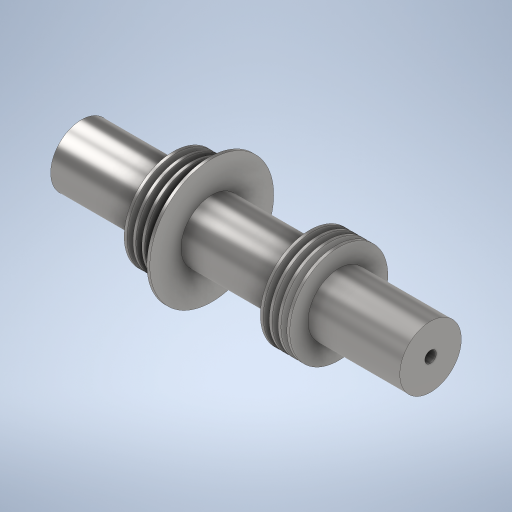
# Autodesk Inventor part: Полный ротор
Saved by Autodesk Inventor 2023 (Build 270158000, 158)
## iProperties
Created: 2023-05-19
Part Number: Полный ротор
Material: Сталь нержавеющая, 440C
Document SubType Name: Modeling
Designer: Roma
Density: 7.75 g/cm^3
Appearance: С умеренной полировкой
Mass: 5.75155e+06 g
Surface Area: 129986 cm^2
Volume: 742136 cm^3
Author: Roma
Autodesk Inventor part; units mm, degrees
ref_plane "YZ Plane" through (0, 0, 0) normal (1, 0, 0) x (0, 1, 0)
ref_plane "XZ Plane" through (0, 0, 0) normal (0, 1, 0) x (-1, 0, 0)
ref_plane "XY Plane" through (0, 0, 0) normal (0, 0, 1) x (1, 0, 0)
derived "Rotor.ipt"
sketch "Эскиз1" plane through (0, 0, 0) normal (0, 0, 1) x (1, 0, 0)
  line L0 (0, 0) -> (3099.5877, 0)
  line L1 (0, 268) -> (800, 268)
  line L2 (800, 268) -> (800, 427.5)
  line L3 (800, 427.5) -> (825.2848, 427.5)
  line L4 (825.2848, 427.5) -> (825.2848, 268)
  line L5 (825.2848, 268) -> (876.9914, 268)
  line L6 (876.9914, 268) -> (876.9914, 427.5)
  line L7 (876.9914, 427.5) -> (902.2762, 427.5)
  line L8 (902.2762, 427.5) -> (902.2762, 268)
  line L9 (902.2762, 268) -> (953.9828, 268)
  line L10 (953.9828, 268) -> (953.9828, 427.5)
  line L11 (953.9828, 427.5) -> (979.2676, 427.5)
  line L12 (979.2676, 427.5) -> (979.2676, 268)
  line L13 (979.2676, 268) -> (1030.9742, 268)
  line L14 (1030.9742, 268) -> (1110.9742, 268)
  line L15 (1110.9742, 268) -> (1110.9742, 540)
  line L16 (1110.9742, 540) -> (1136.259, 540)
  line L17 (1136.259, 540) -> (1136.259, 268)
  line L18 (1136.259, 268) -> (1936.259, 268)
  line L19 (1936.259, 268) -> (1987.9655, 268)
  line L20 (1987.9655, 268) -> (1987.9655, 427.5)
  line L21 (1987.9655, 427.5) -> (2013.2504, 427.5)
  line L22 (2013.2504, 427.5) -> (2013.2504, 268)
  line L23 (2013.2504, 268) -> (2064.9569, 268)
  line L24 (2064.9569, 268) -> (2064.9569, 427.5)
  line L25 (2064.9569, 427.5) -> (2090.2418, 427.5)
  line L26 (2090.2418, 427.5) -> (2090.2418, 268)
  line L27 (2090.2418, 268) -> (2141.9483, 268)
  line L28 (2141.9483, 268) -> (2141.9483, 427.5)
  line L29 (2141.9483, 427.5) -> (2167.2331, 427.5)
  line L30 (2167.2331, 427.5) -> (2167.2331, 268)
  line L31 (2167.2331, 268) -> (2218.9397, 268)
  line L32 (2218.9397, 268) -> (2218.9397, 427.5)
  line L33 (2218.9397, 427.5) -> (2244.2245, 427.5)
  line L34 (2244.2245, 427.5) -> (2244.2245, 268)
  line L35 (2244.2245, 268) -> (3044.2245, 268)
  line L36 (0, 50) -> (3044.2245, 50)
  line L37 (3044.2245, 50) -> (3044.2245, 268)
  line L38 (0, 50) -> (0, 268)
  point P0 (400, 268)
  point P1 (2244.2245, 268)
revolve "Вращение1" add sketch "Эскиз1" angle 360 about axis through (0, 0, 0) along (1, 0, 0)
